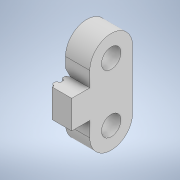
# Autodesk Inventor part: inside belt clamp
Saved by Autodesk Inventor 2022 (Build 260153000, 153)
## iProperties
Created: 2021-12-29
Part Number: inside belt clamp
Material: Generic
Document SubType Name: Modeling
Designer: alexr
Density: 1 g/cm^3
Appearance: Default
Author: alexr
Autodesk Inventor part; units mm, degrees
ref_plane "YZ Plane" through (0, 0, 0) normal (1, 0, 0) x (0, 1, 0)
ref_plane "XZ Plane" through (0, 0, 0) normal (0, 1, 0) x (-1, 0, 0)
ref_plane "XY Plane" through (0, 0, 0) normal (0, 0, 1) x (1, 0, 0)
sketch "Sketch1" plane through (0, 0, 0) normal (1, 0, 0) x (0, 1, 0)
  circle A0 centre (2.3235, 0) radius 2
  circle A1 centre (-9.6765, 0) radius 2
  circle A2 centre (2.3235, 0) radius 4.4
  circle A3 centre (-9.6765, 0) radius 4.4
  line L0 (2.3235, 4.4) -> (-9.6765, 4.4)
  line L1 (-9.6765, -4.4) -> (2.3235, -4.4)
  line L2 (-0.7765, 0) -> (-6.5765, 0)
  line L3 (-6.5765, 0) -> (-6.5765, 8.1162)
  line L4 (-6.5765, 8.1162) -> (-0.7765, 8.1162)
  line L5 (-0.7765, 8.1162) -> (-0.7765, 0)
  point P0 (0, 0)
  point P1 (-0.7765, 4.4)
  point P2 (-6.5765, 4.4)
  dimension "d0" = 4
  dimension "d1" = 4
  dimension "d2" = 12
  dimension "d3" = 8.8
  dimension "d4" = 8.8
  dimension "d5" = 5.8
  dimension "d6" = 3.1
  constraints: 12 end point, 4 centre point, 4 point on circle, 2 coincident, 2 parallel, 2 tangent, 1 horizontal, 1 perpendicular
  measures "d0" diameter of A0
  measures "d1" diameter of A1
  measures "d2" distance of A0.centre A1.centre
  measures "d3" diameter of A2
  measures "d4" diameter of A3
  measures "d5" distance of L3.end L4.end
  measures "d6" distance from line of A1.centre L3
extrude "Extrusion1" add sketch "Sketch1" along normal blind 5
sketch "Sketch2" plane through (0, 0, 0) normal (-1, 0, 0) x (0, 0, 1)
  line L0 (4.4, -0.7765) -> (8.1162, -0.7765) projected
  line L1 (8.1162, -0.7765) -> (-4.6957, -0.7765)
  line L2 (-4.6957, -0.7765) -> (-4.6957, -6.5765)
  line L3 (-4.6957, -6.5765) -> (8.1162, -6.5765)
  line L4 (8.1162, -6.5765) -> (8.1162, -0.7765)
  line L5 (8.1162, -6.5765) -> (4.4, -6.5765) projected
  point P0 (0, 0)
  dimension "d9" = 0
  constraints: 8 end point, 2 parallel, 1 horizontal, 1 perpendicular
  measures "d9" distance between parallel lines of L5 L3
extrude "Extrusion2" cut sketch "Sketch2" against normal blind 1
chamfer "Chamfer1" distance 1 angle 45 2 edges at (0, -0.7765, 0) (0, -6.5765, 0)
sketch "Sketch3" plane through (1, 0, 0) normal (-1, 0, 0) x (0, 0, 1)
  line L0 (-4.4, -6.5765) -> (-4.4, -0.7765) projected
  line L1 (4.4, -6.5765) -> (-4.4, -6.5765) projected
  line L2 (8.1162, -6.5765) -> (4.4, -6.5765) projected
  line L3 (8.1162, -0.7765) -> (8.1162, -6.5765) projected
  line L4 (4.4, -0.7765) -> (8.1162, -0.7765) projected
  line L5 (-4.4, -0.7765) -> (4.4, -0.7765) projected
  line L6 (-4.4, -0.7765) -> (4.4, -0.7765) projected
  line L7 (6.6162, -6.5765) -> (7.6162, -6.5765)
  line L8 (7.6162, -6.5765) -> (7.6162, -0.7765)
  line L9 (7.6162, -0.7765) -> (6.6162, -0.7765)
  line L10 (6.6162, -0.7765) -> (6.6162, -6.5765)
  line L11 (6.6162, -6.5765) -> (7.6162, -0.7765) construction
  line L12 (7.6162, -6.5765) -> (6.6162, -0.7765) construction
  line L13 (4.6162, -0.7765) -> (4.6162, -6.5765)
  line L14 (5.6162, -6.5765) -> (5.6162, -0.7765)
  line L15 (5.6162, -0.7765) -> (4.6162, -0.7765)
  line L16 (4.6162, -6.5765) -> (5.6162, -6.5765)
  line L17 (2.6162, -0.7765) -> (2.6162, -6.5765)
  line L18 (3.6162, -6.5765) -> (3.6162, -0.7765)
  line L19 (3.6162, -0.7765) -> (2.6162, -0.7765)
  line L20 (2.6162, -6.5765) -> (3.6162, -6.5765)
  line L21 (0.6162, -0.7765) -> (0.6162, -6.5765)
  line L22 (1.6162, -6.5765) -> (1.6162, -0.7765)
  line L23 (1.6162, -0.7765) -> (0.6162, -0.7765)
  line L24 (0.6162, -6.5765) -> (1.6162, -6.5765)
  line L25 (-1.3838, -0.7765) -> (-1.3838, -6.5765)
  line L26 (-0.3838, -6.5765) -> (-0.3838, -0.7765)
  line L27 (-0.3838, -0.7765) -> (-1.3838, -0.7765)
  line L28 (-1.3838, -6.5765) -> (-0.3838, -6.5765)
  line L29 (-3.3838, -0.7765) -> (-3.3838, -6.5765)
  line L30 (-2.3838, -6.5765) -> (-2.3838, -0.7765)
  line L31 (-2.3838, -0.7765) -> (-3.3838, -0.7765)
  line L32 (-3.3838, -6.5765) -> (-2.3838, -6.5765)
  point P0 (0, 0)
  point P1 (7.1162, -3.6765)
  point P2 (7.6162, -0.7765)
  point P3 (5.6162, -0.7765)
  point P4 (3.6162, -0.7765)
  point P5 (1.6162, -0.7765)
  point P6 (-0.3838, -0.7765)
  point P7 (-2.3838, -0.7765)
  dimension "d15" = 1
  dimension "d16" = 1
  dimension "d19" = 2
  constraints: 52 end point, 2 horizontal, 2 midpoint, 2 parallel, 1 perpendicular, 1 point on line, 40 other
  measures "d15" distance of L9.end L8.end
  measures "d16" distance from line of L3 point (7.116, -3.676)
  measures "d19" distance of L9.end L13.start
extrude "Extrusion3" add sketch "Sketch3" along normal blind 0.6 contours L29 L5 L30 L1 | L25 L5 L26 L1 | L21 L5 L22 L1 | L17 L5 L18 L1 | L13 L4 L14 L2 | L10 L4 L8 L2
fillet "Fillet1" radius 0.3 24 edges at (1, -3.6765, -3.3838) (0.4, -3.6765, -3.3838) (1, -3.6765, -2.3838) (0.4, -3.6765, -2.3838) (1, -3.6765, -1.3838) (0.4, -3.6765, -1.3838) (1, -3.6765, -0.3838) (0.4, -3.6765, -0.3838) (1, -3.6765, 0.6162) (0.4, -3.6765, 0.6162) (1, -3.6765, 1.6162) (0.4, -3.6765, 1.6162) (1, -3.6765, 2.6162) (0.4, -3.6765, 2.6162) (1, -3.6765, 3.6162) (0.4, -3.6765, 3.6162) (1, -3.6765, 4.6162) (0.4, -3.6765, 4.6162) (1, -3.6765, 5.6162) (0.4, -3.6765, 5.6162) (1, -3.6765, 6.6162) (0.4, -3.6765, 6.6162) (1, -3.6765, 7.6162) (0.4, -3.6765, 7.6162)
equation "\"d4\" = d3"
equation "\"d6\" = -0.5 * d5 + 0.5 * d2"
body "Solid1"
